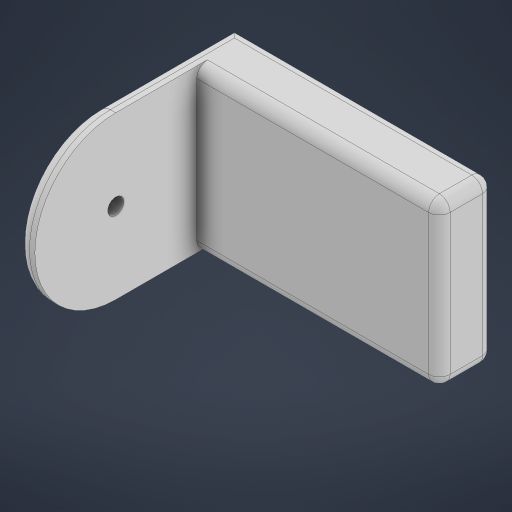
# Autodesk Inventor part: Claw base
Saved by Autodesk Inventor 2023 (Build 270158000, 158)
## iProperties
Created: 2023-04-10
Part Number: Claw base
Material: Generic
Document SubType Name: Modeling
Designer: vatdu
Density: 1 g/cm^3
Appearance: Default
Author: vatdu
Autodesk Inventor part; units mm, degrees
ref_plane "YZ Plane" through (0, 0, 0) normal (1, 0, 0) x (0, 1, 0)
ref_plane "XZ Plane" through (0, 0, 0) normal (0, 1, 0) x (-1, 0, 0)
ref_plane "XY Plane" through (0, 0, 0) normal (0, 0, 1) x (1, 0, 0)
sketch "Sketch1" plane through (0, 0, 0) normal (0, 0, 1) x (1, 0, 0)
  line L0 (0, 0) -> (45, 0)
  line L1 (45, 0) -> (45, 30)
  line L2 (45, 30) -> (0, 30)
  line L3 (0, 30) -> (0, 0)
  dimension "d0" = 45
  dimension "d1" = 30
  constraints: 8 end point, 2 parallel, 1 horizontal, 1 perpendicular
  measures "d0" distance of L2.end L1.end
  measures "d1" distance of L1.end L0.end
extrude "Extrusion1" add sketch "Sketch1" along normal blind 10
sketch "Sketch2" plane through (0, 0, 10) normal (0, 0, 1) x (1, 0, 0)
  line L0 (45, 30) -> (0, 30) projected
  line L1 (0, 30) -> (-3, 30)
  line L2 (-3, 30) -> (-3, 0)
  line L3 (-3, 0) -> (0, 0)
  line L4 (0, 0) -> (0, 30)
  dimension "d4" = 3
  constraints: 8 end point, 2 parallel, 1 horizontal, 1 perpendicular
  measures "d4" distance of L3.end L2.end
extrude "Extrusion2" add sketch "Sketch2" along normal blind 30 and the other way blind 10
fillet "Fillet1" radius 15 2 edges at (-1.5, 30, 40) (-1.5, 0, 40)
sketch "Sketch3" plane through (0, 0, 10) normal (1, 0, 0) x (0, 0, -1)
  arc A0 (-15, 30) -> (-15, 0) centre (-15, 15) ccw projected
  circle A1 centre (-15, 15) radius 1.5
  point P0 (10, 0)
  dimension "d10" = 3
  constraints: 1 centre point, 1 coincident
  measures "d10" diameter of A1
extrude "Extrusion3" cut sketch "Sketch3" against normal blind 30
fillet "Fillet2" radius 2 13 edges at (45, 30, 5) (45, 0, 5) (45, 15, 10) (22.5, 30, 10) (45, 15, 0) (21, 30, 0) (-3, 25.6066, 35.6066) (-3, 15, 40) (-3, 4.3934, 35.6066) (-3, 0, 12.5001) (-3, 30, 12.5001) (21, 0, 0) (22.5, 0, 10)
body "Solid1"
